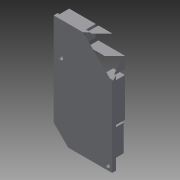
# Autodesk Inventor part: RBC4242
Saved by Autodesk Inventor 2015 (Build 190159000, 159)
## iProperties
Created: 2015-05-04
Part Number: RBC4242
Material: Ogólny
Document SubType Name: Modeling
Designer: Kuba
Density: 1 g/cm^3
Appearance: Domyślna
Author: Kuba
Autodesk Inventor part; units mm, degrees
ref_plane "YZ Plane" through (0, 0, 0) normal (1, 0, 0) x (0, 1, 0)
ref_plane "XZ Plane" through (0, 0, 0) normal (0, 1, 0) x (-1, 0, 0)
ref_plane "XY Plane" through (0, 0, 0) normal (0, 0, 1) x (1, 0, 0)
sketch "Szkic1" plane through (0, 0, 0) normal (0, 1, 0) x (-1, 0, 0)
  line L0 (-22.55, -41.4) -> (22.55, -41.4)
  line L1 (22.55, -41.4) -> (22.55, 41.4)
  line L2 (22.55, 41.4) -> (-22.55, 41.4)
  line L3 (-22.55, 41.4) -> (-22.55, -41.4)
  line L4 (-22.55, -41.4) -> (22.55, 41.4) construction
  line L5 (22.55, -41.4) -> (-22.55, 41.4) construction
  point P0 (0, 0)
  dimension "d0" = 45.1
  dimension "d1" = 82.8
  constraints: 12 end point, 2 midpoint, 2 parallel, 1 horizontal, 1 perpendicular
  measures "d0" distance of L2.end L1.end
  measures "d1" distance of L1.end L0.end
extrude "Wyciągnięcie proste1" add sketch "Szkic1" along normal blind 3
sketch "Szkic2" plane through (0, 3, 0) normal (0, 1, 0) x (1, 0, 0)
  line L0 (22.55, 41.4) -> (-22.55, 41.4) projected
  line L1 (-22.55, 41.4) -> (-22.55, -41.4) projected
  line L2 (-22.55, -41.4) -> (22.55, -41.4) projected
  line L3 (22.55, -41.4) -> (22.55, 41.4) projected
  point P0 (0, 0)
  point P1 (-16.95, -16.1)
  point P2 (19.05, 37.9)
  dimension "d4" = 57.5
  dimension "d5" = 54
  dimension "d6" = 3.5
  dimension "d7" = 36
  measures "d4" distance from line of L0 point (-16.95, -16.1)
  measures "d5" vertical distance of point (-16.95, -16.1) point (19.05, 37.9)
  measures "d6" distance from line of L3 point (19.05, 37.9)
  measures "d7" horizontal distance of point (-16.95, -16.1) point (19.05, 37.9)
hole "Otwór1" at (-16.95, 3, 16.1) at (19.05, 3, -37.9) direction (0, -1, 0) diameter 3.5 end through all
sketch "Szkic3" plane through (0, 3, 0) normal (0, 1, 0) x (1, 0, 0)
  circle A0 centre (-16.95, -16.1) radius 1.75 projected
  circle A1 centre (19.05, 37.9) radius 1.75 projected
  line L0 (22.55, 41.4) -> (-22.55, 41.4) projected
  line L1 (-22.55, 41.4) -> (-22.55, -41.4) projected
  line L2 (-22.55, -41.4) -> (22.55, -41.4) projected
  line L3 (22.55, -41.4) -> (22.55, 41.4) projected
  line L4 (-21.55, -40.9) -> (-1.05, -40.9)
  line L5 (-1.05, -40.9) -> (-1.05, -31.9)
  line L6 (-1.05, -31.9) -> (-21.55, -31.9)
  line L7 (-21.55, -31.9) -> (-21.55, -40.9)
  line L8 (0.95, -40.9) -> (21.45, -40.9)
  line L9 (21.45, -40.9) -> (21.45, -31.9)
  line L10 (21.45, -31.9) -> (0.95, -31.9)
  line L11 (0.95, -31.9) -> (0.95, -40.9)
  line L12 (0.95, -30.9) -> (21.45, -30.9)
  line L13 (21.45, -30.9) -> (21.45, -21.9)
  line L14 (21.45, -21.9) -> (0.95, -21.9)
  line L15 (0.95, -21.9) -> (0.95, -30.9)
  line L16 (20.55, 34.7531) -> (11.55, 34.7531)
  line L17 (11.55, 34.7531) -> (11.55, 14.2531)
  line L18 (11.55, 14.2531) -> (20.55, 14.2531)
  line L19 (20.55, 14.2531) -> (20.55, 34.7531)
  line L20 (10.4919, 34.7531) -> (1.4919, 34.7531)
  line L21 (1.4919, 34.7531) -> (1.4919, 14.2531)
  line L22 (1.4919, 14.2531) -> (10.4919, 14.2531)
  line L23 (10.4919, 14.2531) -> (10.4919, 34.7531)
  line L24 (21.45, 12.0004) -> (12.45, 12.0004)
  line L25 (12.45, 12.0004) -> (12.45, -17.9996)
  line L26 (12.45, -17.9996) -> (21.45, -17.9996)
  line L27 (21.45, -17.9996) -> (21.45, 12.0004)
  line L28 (-20.8756, 23.1013) -> (-11.8756, 23.1013)
  line L29 (-11.8756, 23.1013) -> (-11.8756, 2.6013)
  line L30 (-11.8756, 2.6013) -> (-20.8756, 2.6013)
  line L31 (-20.8756, 2.6013) -> (-20.8756, 23.1013)
  point P0 (0, 0)
  dimension "d15" = 20.5
  dimension "d16" = 9
  dimension "d17" = 1
  dimension "d18" = 0.5
  dimension "d19" = 20.5
  dimension "d20" = 9
  dimension "d21" = 2
  dimension "d22" = 0.5
  dimension "d23" = 20.5
  dimension "d24" = 9
  dimension "d25" = 1
  dimension "d26" = 9
  dimension "d27" = 20.5
  dimension "d28" = 9
  dimension "d29" = 20.5
  dimension "d30" = 9
  dimension "d31" = 30
  dimension "d32" = 9
  dimension "d33" = 20.5
  constraints: 56 end point, 14 parallel, 7 horizontal, 7 perpendicular, 1 point on line
  measures "d15" distance of L6.end L5.end
  measures "d16" distance of L5.end L4.end
  measures "d17" distance between parallel lines of L1 L7
  measures "d18" distance between parallel lines of L2 L4
  measures "d19" distance of L10.end L9.end
  measures "d20" distance of L9.end L8.end
  measures "d21" distance between parallel lines of L5 L11
  measures "d22" distance between parallel lines of L2 L8
  measures "d23" distance of L14.end L13.end
  measures "d24" distance of L13.end L12.end
  measures "d25" distance between parallel lines of L10 L12
  measures "d26" distance of L18.end L17.end
  measures "d27" distance of L17.end L16.end
  measures "d28" distance of L22.end L21.end
  measures "d29" distance of L21.end L20.end
  measures "d30" distance of L26.end L25.end
  measures "d31" distance of L25.end L24.end
  measures "d32" distance of L29.end L30.end
  measures "d33" distance of L28.end L29.end
extrude "Wyciągnięcie proste2" add sketch "Szkic3" along normal blind 8 contours L7 L6 L5 L4 | L11 L10 L9 L8 | L15 L14 L13 L12 | L19 L18 L17 L16 | L23 L22 L21 L20 | L27 L26 L25 L24 | L28 L29 L30 L31
